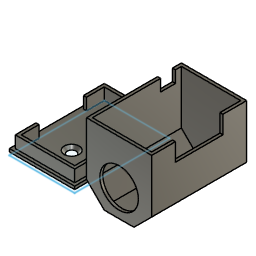
Led Button Casing v6 (Autodesk Fusion 360 design; units mm, degrees)
Autodesk Fusion 360 part; units mm, degrees
sketch "Sketch1" plane through (0, 0, 0) normal (0, 0, 1) x (1, 0, 0)
  line L0 (1, 1) -> (23, 1)
  line L1 (23, 1) -> (23, 33)
  line L2 (23, 33) -> (1, 33)
  line L3 (1, 33) -> (1, 1)
  constraint horizontal L0
  constraint vertical L1
  constraint horizontal L2
  constraint vertical L3
extrude "Extrude10" add sketch "Sketch1" along normal blind 2 and the other way blind -1 makes body 1
sketch "Sketch9" plane through (0, 0, 2) normal (0, 0, 1) x (-1, 0, 0)
  line L0 (-1, -33) -> (-1, -1)
  line L1 (-1, -1) -> (-23, -1)
  line L2 (-23, -1) -> (-23, -33)
  line L3 (-23, -33) -> (-1, -33)
  line L4 (-2, -32) -> (-22, -32)
  line L5 (-22, -32) -> (-22, -2)
  line L6 (-22, -2) -> (-2, -2)
  line L7 (-2, -2) -> (-2, -32)
  line L8 (-3, -31) -> (-21, -31)
  line L9 (-21, -31) -> (-21, -3)
  line L10 (-21, -3) -> (-3, -3)
  line L11 (-3, -3) -> (-3, -31)
  constraint horizontal L4
  constraint vertical L5
  constraint horizontal L6
  constraint vertical L7
  constraint horizontal L8
  constraint vertical L9
  constraint horizontal L10
  constraint vertical L11
extrude "Extrude11" add sketch "Sketch9" along normal blind 4 contours L4 L5 L6 L7 bodies 1
sketch "Sketch10" plane through (0, 0, 0) normal (0, 0, 1) x (1, 0, 0)
  line L0 (31, 1) -> (53, 1)
  line L1 (53, 1) -> (53, 33)
  line L2 (53, 33) -> (31, 33)
  line L3 (31, 33) -> (31, 1)
  line L4 (32, 32) -> (52, 32)
  line L5 (52, 32) -> (52, 2)
  line L6 (52, 2) -> (32, 2)
  line L7 (32, 2) -> (32, 32)
  constraint horizontal L0
  constraint vertical L1
  constraint horizontal L2
  constraint vertical L3
  constraint horizontal L4
  constraint vertical L5
  constraint horizontal L6
  constraint vertical L7
extrude "Extrude12" add sketch "Sketch10" along normal blind 26 and the other way blind -2 separate body makes body 2
extrude "Extrude13" add sketch "Sketch10" along normal blind 26 and the other way blind -25 contours L4 L5 L6 L7 bodies 2
sketch "Sketch11" plane through (0, 1, 0) normal (0, -1, 0) x (1, 0, 0)
  line L0 (31, 2) -> (53, 2)
  line L1 (53, 2) -> (53, 26)
  line L2 (53, 26) -> (31, 26)
  line L3 (31, 26) -> (31, 2)
  circle A0 centre (42, 17) radius 6.5
  dimension "d44" = 13
  measures "d44" diameter of A0
extrude "Extrude14" cut sketch "Sketch11" against normal blind 2 contours A0 bodies 2
chamfer "Chamfer3" distance 5 angle 45 2 edges at (32, 17, 25) (52, 17, 25) on bodies 2
chamfer "Chamfer4" distance 6 angle 45 2 edges at (31, 17, 26) (53, 17, 26) on bodies 2
sketch "Sketch12" plane through (53, 0, 0) normal (1, 0, 0) x (0, 1, 0)
  line L0 (33, 20) -> (1, 20)
  line L1 (1, 20) -> (1, 2)
  line L2 (1, 2) -> (33, 2)
  line L3 (33, 2) -> (33, 20)
  line L4 (30, 2) -> (25, 2)
  line L5 (25, 2) -> (25, 6)
  line L6 (25, 6) -> (30, 6)
  line L7 (30, 6) -> (30, 2)
  constraint horizontal L4
  constraint vertical L5
  constraint horizontal L6
  constraint vertical L7
  constraint coincident L2 L4.start
extrude "Extrude15" cut sketch "Sketch12" against normal blind 2 contours L2 L4 L5 L6 L7 bodies 2
extrude "Extrude16" cut sketch "Sketch12" along normal blind -31 and the other way blind 32 contours L2 L4 L5 L6 L7 bodies 1
sketch "Sketch13" plane through (31, 0, 0) normal (-1, 0, 0) x (0, -1, 0)
  line L0 (-1, 20) -> (-33, 20)
  line L1 (-33, 20) -> (-33, 2)
  line L2 (-33, 2) -> (-1, 2)
  line L3 (-1, 2) -> (-1, 20)
  line L4 (-25, 2) -> (-9, 2)
  line L5 (-9, 2) -> (-9, 8)
  line L6 (-9, 8) -> (-25, 8)
  line L7 (-25, 8) -> (-25, 2)
  constraint horizontal L4
  constraint vertical L5
  constraint horizontal L6
  constraint vertical L7
  constraint coincident L2 L4.start
extrude "Extrude17" cut sketch "Sketch13" against normal blind 2 contours L2 L4 L5 L6 L7 bodies 2
extrude "Extrude18" cut sketch "Sketch13" along normal blind 29 and the other way blind -28 contours L2 L4 L5 L6 L7 bodies 1
move_body "Move1" bodies 2 to x (-1, 0, 0) y (0, 1, 0) z (0, 0, -1) at (80, 0, 26)
sketch "Sketch14" plane through (0, 0, 2) normal (0, 0, 1) x (-1, 0, 0)
  line L0 (-22, -25) -> (-22, -2)
  line L1 (-22, -2) -> (-2, -2)
  line L2 (-2, -2) -> (-2, -9)
  line L3 (-1, -33) -> (-1, -1)
  line L4 (-1, -1) -> (-23, -1)
  line L5 (-23, -1) -> (-23, -33)
  line L6 (-23, -33) -> (-1, -33)
  line L7 (-2, -32) -> (-22, -32)
  circle A0 centre (-12, -11) radius 1.5
  circle A1 centre (-12, -24) radius 1.5
  line L8 (-22, -30) -> (-21, -30)
  line L9 (-21, -30) -> (-21, -31)
  line L10 (-21, -31) -> (-3, -31)
  line L11 (-3, -9) -> (-3, -3)
  line L12 (-3, -3) -> (-21, -3)
  line L13 (-21, -3) -> (-21, -25)
  line L14 (-21, -25) -> (-22, -25)
  line L15 (-2, -9) -> (-3, -9)
  line L16 (-3, -25) -> (-2, -25)
  line L17 (-2, -25) -> (-2, -32)
  line L18 (-22, -32) -> (-22, -30)
  line L19 (-3, -31) -> (-3, -25)
extrude "Extrude19" cut sketch "Sketch14" against normal blind 2 contours A0 | A1 bodies 1
chamfer "Chamfer5" distance 1 angle 45 2 edges at (13.3985, 23.4576, 2) (13.3985, 10.4576, 2) on bodies 1
